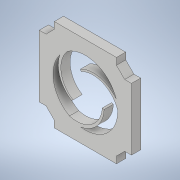
# Autodesk Inventor part: 20_Cube_Insert_Holder-okular+flashlight_v2
Saved by Autodesk Inventor 2022 (Build 260153000, 153)
## iProperties
Created: 2019-07-24
Part Number: 20_Cube_Insert_Holder-okular+flashlight_v2
Material: Generic
Document SubType Name: Modeling
Designer: marsikovabarbora
Density: 1 g/cm^3
Appearance: Default
Author: marsikovabarbora
Autodesk Inventor part; units mm, degrees
ref_plane "YZ Plane" through (0, 0, 0) normal (1, 0, 0) x (0, 1, 0)
ref_plane "XZ Plane" through (0, 0, 0) normal (0, 1, 0) x (-1, 0, 0)
ref_plane "XY Plane" through (0, 0, 0) normal (0, 0, 1) x (1, 0, 0)
sketch "Sketch1" plane through (0, 0, 0) normal (0, 0, 1) x (1, 0, 0)
  line L0 (21.5871, 13.6345) -> (17.0871, 18.1345) projected
  line L1 (17.0871, 18.1345) -> (-16.7129, 18.1345) projected
  line L2 (-16.7129, 18.1345) -> (-21.2129, 13.6345) projected
  line L3 (-21.0966, 13.6345) -> (-21.0966, -20.1655) projected
  line L4 (21.4709, -20.1655) -> (21.4709, 13.6345) projected
  line L5 (21.4709, -20.1655) -> (17.0871, -24.4078) projected
  line L6 (-16.7129, -24.4078) -> (17.0871, -24.4078) projected
  line L7 (-16.7129, -24.4078) -> (-21.0966, -20.1655) projected
  line L8 (-24.7129, -28.1655) -> (-24.7129, 13.6345) construction
  line L9 (25.0871, -28.1655) -> (-24.7129, -28.1655) construction
  line L10 (25.0871, -28.1655) -> (25.0871, 13.6345) construction
  line L11 (17.0871, 21.6345) -> (-16.7129, 21.6345) construction
  arc A0 (-2.2513, -20.5948) -> (10.3132, -6.1041) centre (-5.0595, -5.4673) ccw
  line L12 (9.3473, -5.8453) -> (10.3132, -6.1041)
  arc A1 (-8.4319, -18.4958) -> (9.3473, -5.8453) centre (-4.6285, -5.0223) ccw
  arc A2 (-13.5651, 7.557) -> (-7.2153, -10.699) centre (0.9173, 2.362) ccw
  line L13 (-6.5082, -9.9918) -> (-7.2153, -10.699)
  arc A3 (-9.3703, 11.3941) -> (-6.5082, -9.9918) centre (0.9045, 1.8847) ccw
  arc A4 (16.8103, 2.2043) -> (-2.4098, 6.4971) centre (4.6233, -7.1873) ccw
  line L14 (-2.1509, 5.5312) -> (-2.4098, 6.4971)
  arc A5 (17.6816, -2.8271) -> (-2.1509, 5.5312) centre (4.2873, -6.9006) ccw
  line L15 (0.1871, -36.5255) -> (0.1871, 21.9945)
  line L16 (14.6206, -3.2655) -> (-14.2825, -3.2655) construction
  line L17 (-21.0552, -20.0655) -> (-16.6129, -24.5078)
  line L18 (-16.6129, -24.5078) -> (-16.6129, -28.1655)
  line L19 (-16.6129, -28.1655) -> (16.9871, -28.1655)
  line L20 (16.9871, -28.1655) -> (16.9871, -24.5078)
  line L21 (16.9871, -24.5078) -> (21.4295, -20.0655)
  line L22 (25.0871, -20.0655) -> (21.4295, -20.0655)
  line L23 (25.0871, 13.5345) -> (25.0871, -20.0655)
  line L24 (21.4295, 13.5345) -> (25.0871, 13.5345)
  line L25 (21.4295, 13.5345) -> (16.9871, 17.9768)
  line L26 (16.9871, 17.9768) -> (16.9871, 21.6345)
  line L27 (16.9871, 21.6345) -> (-16.6129, 21.6345)
  line L28 (-16.6129, 21.6345) -> (-16.6129, 17.9768)
  line L29 (-16.6129, 17.9768) -> (-21.0552, 13.5345)
  line L30 (-24.7129, 13.5345) -> (-21.0552, 13.5345)
  line L31 (-24.7129, -20.0655) -> (-24.7129, 13.5345)
  line L32 (-21.0552, -20.0655) -> (-24.7129, -20.0655)
  circle A6 centre (0.1871, -3.2655) radius 17.5
  point P0 (0, 0)
  point P1 (14.2, -44.8454)
  point P2 (9.8303, -5.9747)
  point P3 (0, 0)
  point P4 (16.9871, 19.8057)
  dimension "d48" = 35
  dimension "d49" = 1
  dimension "d50" = 1
  dimension "d51" = 1
  constraints: 42 end point, 18 point on circle, 8 horizontal, 7 centre point, 6 vertical, 2 midpoint, 1 coincident, 8 other
  measures "d48" diameter of A6
  measures "d49" distance of L13.start L13.end
  measures "d50" distance of L14.start L14.end
  measures "d51" distance of L12.start L12.end
extrude "Extrusion1" add sketch "Sketch1" along normal blind 5 contours L26 L25 L24 L4 L22 L21 L6 L15 A6 L1 | L1 L15 L27 L26 | L15 A6 L6 L17 L32 L3 L30 L29 L28 L1 | L1 L28 L27 L15 | L15 A5 L14 A4 | A4 A6 A5 L15 | A3 L13 A2 A6 | L24 L23 L22 L4 | L3 L32 L31 L30 | L15 A0 A6 A1 | A1 L12 A0 L15 | L21 L20 L19 L15 L6 | L15 L19 L18 L17 L6
body "Solid1"
